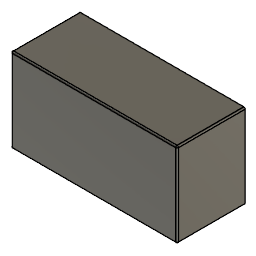
imu_box_v3 (Autodesk Fusion 360 design; units mm, degrees)
Autodesk Fusion 360 part; units mm, degrees
note: some values were not read from the file. Set by a fixed rule: which sketch regions a step uses.
sketch "Sketch1" plane through (0, 0, 0) normal (0, 1, 0) x (1, 0, 0)
  line L0 (0, 0) -> (55, 0)
  line L1 (55, 0) -> (55, -25)
  line L2 (55, -25) -> (0, -25)
  line L3 (0, -25) -> (0, 0)
  line L4 (58, 3) -> (58, -28)
  line L5 (58, -28) -> (-3, -28)
  line L6 (-3, -28) -> (-3, 3)
  line L7 (-3, 3) -> (58, 3)
  dimension "d1" = 55
  dimension "d2" = 25
  dimension "d3" = -3
  constraint horizontal L0
  constraint vertical L1
  constraint horizontal L2
  constraint vertical L3
  constraint coincident L0.start L3.end
  measures "d1" distance of L1.end L2.end
  measures "d2" distance of L0.end L1.end
extrude "Extrude1" add sketch "Sketch1" along normal blind 25 makes body 1
extrude "Extrude2" add sketch "Sketch1" along normal blind 3 contours L0 L1 L2 L3 bodies 1
ref_plane "WorkPlane1" through (27.5, 12.5, 12.5) normal (0, 0, 1) x (1, 0, 0)
ref_plane "WorkPlane2" through (27.5, 12.5, 12.5) normal (1, 0, 0) x (0, 0, -1)
sketch "Sketch3" plane through (27.5, 0, 0) normal (1, 0, 0) x (0, 1, 0)
  line L0 (25, 28) -> (0, 28)
  line L1 (0, 28) -> (0, -3)
  line L2 (0, -3) -> (25, -3)
  line L3 (25, -3) -> (25, 0)
  line L4 (25, 0) -> (3, 0)
  line L5 (3, 0) -> (3, 25)
  line L6 (3, 25) -> (25, 25)
  line L7 (25, 25) -> (25, 28)
  circle A0 centre (19.5448, 25) radius 0.75
  circle A1 centre (19.5448, 25) radius 0.85
  line L8 (25, -3) -> (27, -3)
  line L9 (27, -3) -> (27, 28)
  line L10 (27, 28) -> (25, 28)
  line L11 (25, 25) -> (25, 0)
  arc A2 (18.8036, 24.8855) -> (25, 16.7817) centre (26.1363, 24.0714) ccw
  arc A3 (20.2801, 24.8524) -> (25, 24.3618) centre (22.7071, 25.2525) ccw
  line L12 (25.7, 12.5) -> (-0.7, 12.5)
  arc A4 (25, 0.6382) -> (20.2801, 0.1476) centre (22.7071, -0.2525) ccw
  arc A5 (20.2801, 0.1476) -> (19.4995, -1.0498) centre (22.5513, -2.1863) ccw
  arc A6 (25, 8.2183) -> (18.8036, 0.1145) centre (26.1363, 0.9286) ccw
  circle A7 centre (19.5448, 0) radius 0.85
  circle A8 centre (19.5448, 0) radius 0.75
  dimension "d8" = 1.5
  dimension "d9" = 0.1
  constraint coincident L6 A0.centre
  constraint coincident L2.end L3.start
  constraint perpendicular L3 L8
  constraint perpendicular L8 L9
  constraint coincident L0.start L7.end
  constraint coincident L6.end L7.start
  constraint coincident L3.end L4.start
  constraint coincident L11 A2.end
  constraint coincident L11 A3.end
  constraint symmetric A0 L12 A8
  constraint symmetric A1 L12 A7
  constraint symmetric A2.end L12 A6.start
  constraint symmetric A2 L12 A6
  constraint symmetric A3.end L12 A4.start
  constraint symmetric A3 L12 A4
  constraint symmetric A3.start L12 A4.end
  constraint symmetric A2.start L12 A6.end
  constraint coincident A0 A2.start
  constraint coincident A0 A3.start
  measures "d8" diameter of A0
extrude "Extrude3" cut sketch "Sketch3" against normal up to surface (55 mm away) from surface at 27.5 contours L6 A0 A1 A3 | L6 A0 A1 | L6 A0 | L6 A0 | L6 A0 A1 A2 | L4 A5 A7 A8 | L4 A5 A7 A8 | L4 A5 A8 | L4 A5 A8 | L4 A5 A8 | L4 A5 A8 bodies 1
extrude "Extrude4" add sketch "Sketch3" along normal mid plane 61 separate body contours L3 L7 L8 L9 L10 L11 makes body 2
extrude "Extrude5" add sketch "Sketch3" along normal blind 4 from surface at 10 contours A1 L11 A2 A3 | L6 A0 | L6 A0 | A0 A1 A2 A3 | L11 A4 A6 A7 | L4 A5 A8 | L4 A5 A8 | A4 A6 A7 A8 | L4 A5 A8 | L4 A5 A8 bodies 2
extrude "Extrude6" add sketch "Sketch3" along normal blind 4 from surface at -10 contours A1 L11 A2 A3 | L6 A0 | L6 A0 | A0 A1 A2 A3 | L11 A4 A6 A7 | L4 A5 A8 | L4 A5 A8 | A4 A6 A7 A8 | L4 A5 A8 | L4 A5 A8 bodies 2
fillet "Fillet1" radius 1 2 edges at (27.5, 20.3948, 25) (27.5, 20.3948, 0) on bodies 1
fillet "Fillet2" radius 1 2 edges at (27.5, 25, 0) (27.5, 25, 25) on bodies 1
fillet "Fillet2" radius 0.5 2 edges at (55, 25, 12.5) (0, 25, 12.5) on bodies 1
fillet "Fillet3" radius 0.5 4 edges at (27.5, 27, 28) (27.5, 27, -3) (-3, 27, 12.5) (58, 27, 12.5) on bodies 2
fillet "Fillet4" radius 0.5 16 edges at (58, 12.5, -3) (58, 12.5, 28) (-3, 12.5, -3) (-3, 12.5, 28) (-3, 0, 12.5) (27.5, 0, -3) (58, 0, 12.5) (27.5, 0, 28) (58, 25.75, -3) (57.8536, 26.8536, -2.8536) (57.8536, 26.8536, 27.8536) (58, 25.75, 28) (-2.8536, 26.8536, -2.8536) (-3, 25.75, -3) (-3, 25.75, 28) (-2.8536, 26.8536, 27.8536) on bodies 1 2
sketch "Sketch6" plane through (0, 25, 0) normal (0, -1, 0) x (1, 0, 0)
  line L0 (17.5, 8.2183) -> (21.5, 8.2183)
  line L1 (21.5, 8.2183) -> (21.5, 0.6382)
  line L2 (21.5, 0.6382) -> (17.5, 0.6382)
  line L3 (17.5, 0.6382) -> (17.5, 8.2183)
  line L4 (21.5, 16.7817) -> (17.5, 16.7817)
  line L5 (17.5, 16.7817) -> (17.5, 24.3618)
  line L6 (17.5, 24.3618) -> (21.5, 24.3618)
  line L7 (21.5, 24.3618) -> (21.5, 16.7817)
  line L8 (41.5, 16.7817) -> (37.5, 16.7817)
  line L9 (37.5, 16.7817) -> (37.5, 24.3618)
  line L10 (37.5, 24.3618) -> (41.5, 24.3618)
  line L11 (41.5, 24.3618) -> (41.5, 16.7817)
  line L12 (37.5, 8.2183) -> (41.5, 8.2183)
  line L13 (41.5, 8.2183) -> (41.5, 0.6382)
  line L14 (41.5, 0.6382) -> (37.5, 0.6382)
  line L15 (37.5, 0.6382) -> (37.5, 8.2183)
  arc A0 (-2.5, 28) -> (-3, 27.5) centre (-2.5, 27.5) ccw
  line L16 (-3, 27.5) -> (-3, -2.5)
  arc A1 (-3, -2.5) -> (-2.5, -3) centre (-2.5, -2.5) ccw
  line L17 (-2.5, -3) -> (57.5, -3)
  arc A2 (57.5, -3) -> (58, -2.5) centre (57.5, -2.5) ccw
  line L18 (58, -2.5) -> (58, 27.5)
  arc A3 (58, 27.5) -> (57.5, 28) centre (57.5, 27.5) ccw
  line L19 (57.5, 28) -> (-2.5, 28)
  line L20 (55, 25) -> (0, 25)
  line L21 (0, 25) -> (0, 0)
  line L22 (0, 0) -> (55, 0)
  line L23 (55, 0) -> (55, 25)
  line L24 (0, 10) -> (2, 10)
  line L25 (2, 10) -> (2, 15)
  line L26 (2, 15) -> (0, 15)
  line L27 (0, 10) -> (0, 15)
  line L28 (0, 10) -> (0, 15)
  line L29 (55, 15) -> (53, 15)
  line L30 (53, 15) -> (53, 10)
  line L31 (53, 10) -> (55, 10)
  line L32 (55, 15) -> (55, 10)
  constraint coincident L21 L24.start
  constraint perpendicular L21 L24
  constraint perpendicular L24 L25
  constraint coincident L21 L26.end
  constraint perpendicular L21 L26
  constraint coincident L23 L29.start
  constraint perpendicular L23 L29
  constraint perpendicular L29 L30
  constraint coincident L23 L31.end
  constraint perpendicular L23 L31
extrude "Extrude7" add sketch "Sketch6" along normal blind 2 contours L23 L29 L30 L31 L32 bodies 2
extrude "Extrude8" add sketch "Sketch6" along normal blind 2 contours L21 L24 L25 L26 L27 L28 bodies 2
sketch "Sketch7" plane through (0, 0, 0) normal (-1, 0, 0) x (0, -1, 0)
  line L0 (-25, 15) -> (-25, 10)
  line L1 (-25, 10) -> (-23, 10)
  line L2 (-23, 10) -> (-23, 15)
  line L3 (-23, 15) -> (-25, 15)
move_face "OffsetFaces1" offset -0.2 1 faces at (0, 24.3333, 13.3333) on bodies 2
move_face "OffsetFaces2" offset -0.2 1 faces at (55, 24.3333, 11.6667) on bodies 2
hidden bodies 2
